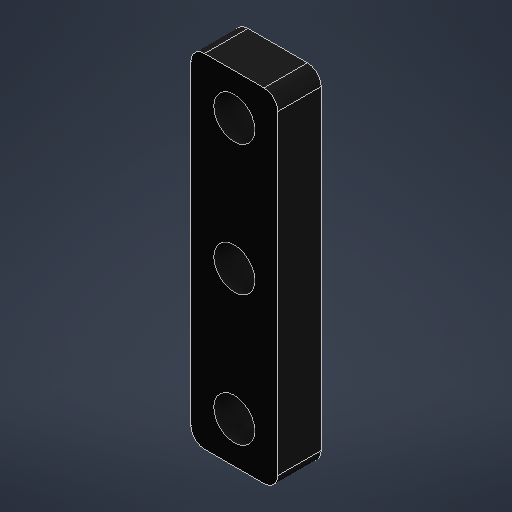
# Autodesk Inventor part: INTAKE_HARDSTOPS
Saved by Autodesk Inventor 2026.2 (Build 302298010, 298A)
## iProperties
Created: 2026-04-02
Part Number: INTAKE_HARDSTOPS
Material: 3D Print Material - chopped carbon Nylon12 (preferred)
Document SubType Name: Modeling
Designer: 4aida
Density: 1.05184 g/cm^3
Appearance: Black
Author: 4aida
Autodesk Inventor part; units mm, degrees
ref_plane "YZ Plane" through (0, 0, 0) normal (1, 0, 0) x (0, 1, 0)
ref_plane "XZ Plane" through (0, 0, 0) normal (0, 1, 0) x (-1, 0, 0)
ref_plane "XY Plane" through (0, 0, 0) normal (0, 0, 1) x (1, 0, 0)
sketch "Sketch1" plane through (0, 0, 0) normal (0, 0, 1) x (1, 0, 0)
  line L0 (6.35, -25.05) -> (-6.35, -25.05)
  line L1 (-6.35, -25.05) -> (-6.35, 25.05)
  line L2 (-6.35, 25.05) -> (6.35, 25.05)
  line L3 (6.35, 25.05) -> (6.35, -25.05)
  line L4 (6.35, -25.05) -> (-6.35, 25.05) construction
  line L5 (-6.35, -25.05) -> (6.35, 25.05) construction
  circle A0 centre (0, 19.05) radius 3
  circle A1 centre (0, 0) radius 3
  circle A2 centre (0, -19.05) radius 3
  dimension "d0" = 50.1
  dimension "d1" = 19.05
  dimension "d2" = 19.05
  dimension "d3" = 6
  dimension "d4" = 12.7
  constraints: 12 end point, 3 centre point, 2 equal radius, 2 midpoint, 2 parallel, 2 vertical alignment, 1 coincident, 1 horizontal, 1 perpendicular
  measures "d0" distance of L2.end L0.start
  measures "d1" distance of point (0, 0) A0.centre
  measures "d2" distance of A2.centre point (0, 0)
  measures "d3" diameter of A1
  measures "d4" distance of L1.end L2.end
extrude "Extrusion1" add sketch "Sketch1" along normal blind 6.35
fillet "Fillet1" radius 2 4 edges at (6.35, 25.05, 3.175) (-6.35, 25.05, 3.175) (6.35, -25.05, 3.175) (-6.35, -25.05, 3.175)
equation "\"d2\" = d1"
body "Solid1"
